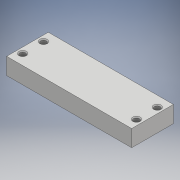
# Autodesk Inventor part: soporte_rueca
Saved by Autodesk Inventor 2018 (Build 220112000, 112)
## iProperties
Created: 2019-06-12
Part Number: soporte_rueca
Material: Genérico
Document SubType Name: Modeling
Designer: Usuario
Density: 1 g/cm^3
Appearance: Valor por defecto
Author: Usuario
Autodesk Inventor part; units mm, degrees
ref_plane "YZ Plane" through (0, 0, 0) normal (1, 0, 0) x (0, 1, 0)
ref_plane "XZ Plane" through (0, 0, 0) normal (0, 1, 0) x (-1, 0, 0)
ref_plane "XY Plane" through (0, 0, 0) normal (0, 0, 1) x (1, 0, 0)
sketch "Boceto1" plane through (0, 0, 0) normal (0, 0, 1) x (1, 0, 0)
  line L0 (3.3269, 0.8317) -> (3.3269, 50.8317)
  line L1 (3.3269, 50.8317) -> (153.3269, 50.8317)
  line L2 (153.3269, 50.8317) -> (153.3269, 0.8317)
  line L3 (153.3269, 0.8317) -> (3.3269, 0.8317)
  point P0 (0, 0)
  dimension "d0" = 150
  dimension "d1" = 50
  constraints: 8 end point, 3 perpendicular, 1 vertical
  measures "d0" distance of L0.end L1.end
  measures "d1" distance of L0.start L0.end
extrude "Extrusión1" add sketch "Boceto1" along normal mid plane 20
sketch "Boceto3" plane through (0, 0, 10) normal (0, 0, 1) x (1, 0, 0)
  circle A0 centre (146.5928, 38.3317) radius 3.5
  circle A1 centre (146.5928, 13.3317) radius 3.5
  line L0 (3.3269, 50.8317) -> (153.3269, 50.8317) projected
  circle A2 centre (146.5928, 38.3317) radius 4.5
  circle A3 centre (146.5928, 13.3317) radius 4.5
  line L1 (153.3269, 50.8317) -> (3.3269, 50.8317) projected
  circle A4 centre (10.0609, 38.3317) radius 3.5
  circle A5 centre (10.0609, 13.3317) radius 3.5
  circle A6 centre (10.0609, 38.3317) radius 4.5
  circle A7 centre (10.0609, 13.3317) radius 4.5
  point P0 (0, 0)
  dimension "d8" = 7
  dimension "d9" = 7
  dimension "d10" = 25
  dimension "d11" = 12.5
  dimension "d12" = 9
  dimension "d13" = 9
  constraints: 8 centre point, 4 coincident
  measures "d8" diameter of A0
  measures "d9" diameter of A1
  measures "d10" distance of A1.centre A0.centre
  measures "d11" distance from line of A0.centre L0
  measures "d12" diameter of A3
  measures "d13" diameter of A2
hole "Agujero1" at (10.0609, 38.3317, 10) at (10.0609, 13.3317, 10) at (146.5928, 38.3317, 10) at (146.5928, 13.3317, 10) direction (0, 0, -1) diameter 7 depth 40 countersink diameter 9 countersink angle 82
